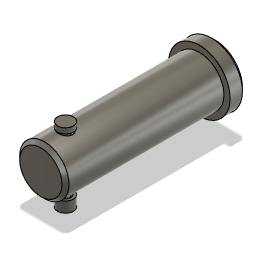
0.174.2818 - Axe d'articulation avec tête 14-45 type B (Autodesk Fusion 360 design; units mm, degrees)
Autodesk Fusion 360 part; units mm, degrees
sketch "Sketch1" plane through (0, 0, 0) normal (0, 0, 1) x (1, 0, 0)
  circle A0 centre (0, 0) radius 7
  dimension "d1" = 14
  constraint coincident A0.centre origin
  measures "d1" diameter of A0
extrude "Extrude1" add sketch "Sketch1" along normal blind 45 makes body 1
chamfer "Chamfer1" distance 1 angle 45 1 edges at (-6.5263, -2.5313, 45) on bodies 1
sketch "Sketch2" plane through (0, 0, 0) normal (0, 0, -1) x (-1, 0, 0)
  circle A0 centre (0, 0) radius 7
  circle A1 centre (0, 0) radius 8.75
  dimension "d5" = 17.5
  constraint coincident A0.centre A1.centre
  measures "d5" diameter of A1
extrude "Extrude2" add sketch "Sketch2" along normal blind 4.5 contours A0 | A1 bodies 1
chamfer "Chamfer2" distance 1 angle 45 1 edges at (8.1579, -3.1641, -4.5) on bodies 1
sketch "Sketch3" plane through (0, 0, 0) normal (0, 1, 0) x (1, 0, 0)
  line L0 (-7, -44) -> (7, -44) construction
  line L1 (-7, -38) -> (7, -38) construction
  line L2 (0, -44) -> (0, -38) construction
  circle A0 centre (0, -38) radius 2
  dimension "d9" = 6
  dimension "d10" = 4
  constraint midpoint L0 L2.start
  constraint midpoint L1 L2.end
  constraint perpendicular L1 L2
  constraint coincident L2.end A0.centre
  measures "d10" diameter of A0
extrude "Extrude3" cut sketch "Sketch3" along normal through all and the other way through all bodies 1
sketch "Sketch4" plane through (0, 0, 0) normal (0, 1, 0) x (1, 0, 0)
  spline S0 degree 3 poles (1.5, -38) (1.5, -37.8138) (1.4604, -37.6052) (1.385, -37.424) (1.3095, -37.2425) (1.1904, -37.0691) (1.0607, -36.9393) (0.931, -36.8096) (0.7575, -36.6905) (0.576, -36.615) (0.3947, -36.5396) (0.186, -36.5) (0, -36.5) (-0.186, -36.5) (-0.3947, -36.5396) (-0.576, -36.615) (-0.7575, -36.6905) (-0.931, -36.8096) (-1.0607, -36.9393) (-1.1904, -37.0691) (-1.3095, -37.2425) (-1.385, -37.424) (-1.4604, -37.6052) (-1.5, -37.8138) (-1.5, -38) (-1.5, -38.1862) (-1.4604, -38.3948) (-1.385, -38.576) (-1.3095, -38.7575) (-1.1904, -38.9309) (-1.0607, -39.0607) (-0.931, -39.1904) (-0.7575, -39.3095) (-0.576, -39.385) (-0.3947, -39.4604) (-0.186, -39.5) (0, -39.5) (0.186, -39.5) (0.3947, -39.4604) (0.576, -39.385) (0.7575, -39.3095) (0.931, -39.1904) (1.0607, -39.0607) (1.1904, -38.9309) (1.3095, -38.7575) (1.385, -38.576) (1.4604, -38.3948) (1.5, -38.1862) (1.5, -38) knots 0.60776 0.60776 0.60776 0.60776 0.683748 0.683748 0.683748 0.759735 0.759735 0.759735 0.835688 0.835688 0.835688 0.91164 0.91164 0.91164 0.987593 0.987593 0.987593 1.063545 1.063545 1.063545 1.139533 1.139533 1.139533 1.21552 1.21552 1.21552 1.291508 1.291508 1.291508 1.367496 1.367496 1.367496 1.443448 1.443448 1.443448 1.5194 1.5194 1.5194 1.595353 1.595353 1.595353 1.671305 1.671305 1.671305 1.747293 1.747293 1.747293 1.82328 1.82328 1.82328 1.82328
  spline S1 degree 3 poles (-2, -38) (-2, -37.7473) (-1.9492, -37.4788) (-1.7447, -36.9865) (-1.591, -36.7626) (-1.2375, -36.409) (-1.0135, -36.2553) (-0.5211, -36.0508) (-0.2526, -36) (0.2526, -36) (0.5211, -36.0508) (1.0135, -36.2553) (1.2375, -36.409) (1.591, -36.7626) (1.7447, -36.9865) (1.9492, -37.4788) (2, -37.7473) (2, -38.2527) (1.9492, -38.5212) (1.7447, -39.0135) (1.591, -39.2374) (1.2375, -39.591) (1.0135, -39.7447) (0.5211, -39.9492) (0.2526, -40) (-0.2526, -40) (-0.5211, -39.9492) (-1.0135, -39.7447) (-1.2375, -39.591) (-1.591, -39.2374) (-1.7447, -39.0135) (-1.9492, -38.5212) (-2, -38.2527) (-2, -38) knots 0 0 0 0 0.075804 0.075804 0.151609 0.151609 0.227394 0.227394 0.30318 0.30318 0.378966 0.378966 0.454752 0.454752 0.530556 0.530556 0.60636 0.60636 0.682165 0.682165 0.757969 0.757969 0.833755 0.833755 0.909541 0.909541 0.985326 0.985326 1.061112 1.061112 1.136916 1.136916 1.212721 1.212721 1.212721 1.212721
  line L0 (0, -68) -> (8.4815, -68)
  constraint horizontal L0
extrude "Extrude4" add sketch "Sketch4" along normal blind 9 and the other way blind 12 separate body contours S0 makes body 2
sketch "Sketch5" plane through (0, 9, 0) normal (0, 1, 0) x (-1, 0, 0)
  spline S0 degree 3 poles (1.5, -38) (1.5, -37.8138) (1.4604, -37.6052) (1.385, -37.424) (1.3095, -37.2425) (1.1904, -37.0691) (1.0607, -36.9393) (0.931, -36.8096) (0.7575, -36.6905) (0.576, -36.615) (0.3947, -36.5396) (0.186, -36.5) (0, -36.5) (-0.186, -36.5) (-0.3947, -36.5396) (-0.576, -36.615) (-0.7575, -36.6905) (-0.931, -36.8096) (-1.0607, -36.9393) (-1.1904, -37.0691) (-1.3095, -37.2425) (-1.385, -37.424) (-1.4604, -37.6052) (-1.5, -37.8138) (-1.5, -38) (-1.5, -38.1862) (-1.4604, -38.3948) (-1.385, -38.576) (-1.3095, -38.7575) (-1.1904, -38.9309) (-1.0607, -39.0607) (-0.931, -39.1904) (-0.7575, -39.3095) (-0.576, -39.385) (-0.3947, -39.4604) (-0.186, -39.5) (0, -39.5) (0.186, -39.5) (0.3947, -39.4604) (0.576, -39.385) (0.7575, -39.3095) (0.931, -39.1904) (1.0607, -39.0607) (1.1904, -38.9309) (1.3095, -38.7575) (1.385, -38.576) (1.4604, -38.3948) (1.5, -38.1862) (1.5, -38) knots 0.60776 0.60776 0.60776 0.60776 0.683748 0.683748 0.683748 0.759735 0.759735 0.759735 0.835688 0.835688 0.835688 0.91164 0.91164 0.91164 0.987593 0.987593 0.987593 1.063545 1.063545 1.063545 1.139533 1.139533 1.139533 1.21552 1.21552 1.21552 1.291508 1.291508 1.291508 1.367496 1.367496 1.367496 1.443448 1.443448 1.443448 1.5194 1.5194 1.5194 1.595353 1.595353 1.595353 1.671305 1.671305 1.671305 1.747293 1.747293 1.747293 1.82328 1.82328 1.82328 1.82328
  spline S1 degree 3 poles (-1.5, 38) (-1.5, 37.8138) (-1.4604, 37.6052) (-1.385, 37.424) (-1.3095, 37.2425) (-1.1904, 37.0691) (-1.0607, 36.9393) (-0.931, 36.8096) (-0.7575, 36.6905) (-0.576, 36.615) (-0.3947, 36.5396) (-0.186, 36.5) (0, 36.5) (0.186, 36.5) (0.3947, 36.5396) (0.576, 36.615) (0.7575, 36.6905) (0.931, 36.8096) (1.0607, 36.9393) (1.1904, 37.0691) (1.3095, 37.2425) (1.385, 37.424) (1.4604, 37.6052) (1.5, 37.8138) (1.5, 38) (1.5, 38.1862) (1.4604, 38.3948) (1.385, 38.576) (1.3095, 38.7575) (1.1904, 38.9309) (1.0607, 39.0607) (0.931, 39.1904) (0.7575, 39.3095) (0.576, 39.385) (0.3947, 39.4604) (0.186, 39.5) (0, 39.5) (-0.186, 39.5) (-0.3947, 39.4604) (-0.576, 39.385) (-0.7575, 39.3095) (-0.931, 39.1904) (-1.0607, 39.0607) (-1.1904, 38.9309) (-1.3095, 38.7575) (-1.385, 38.576) (-1.4604, 38.3948) (-1.5, 38.1862) (-1.5, 38) knots 0.60776 0.60776 0.60776 0.60776 0.683748 0.683748 0.683748 0.759735 0.759735 0.759735 0.835688 0.835688 0.835688 0.91164 0.91164 0.91164 0.987593 0.987593 0.987593 1.063545 1.063545 1.063545 1.139533 1.139533 1.139533 1.21552 1.21552 1.21552 1.291508 1.291508 1.291508 1.367496 1.367496 1.367496 1.443448 1.443448 1.443448 1.5194 1.5194 1.5194 1.595353 1.595353 1.595353 1.671305 1.671305 1.671305 1.747293 1.747293 1.747293 1.82328 1.82328 1.82328 1.82328 construction
  spline S2 degree 3 poles (-1.5, 38) (-1.5, 38.1862) (-1.4604, 38.3948) (-1.385, 38.576) (-1.3095, 38.7575) (-1.1904, 38.9309) (-1.0607, 39.0607) (-0.931, 39.1904) (-0.7575, 39.3095) (-0.576, 39.385) (-0.3947, 39.4604) (-0.186, 39.5) (0, 39.5) (0.186, 39.5) (0.3947, 39.4604) (0.576, 39.385) (0.7575, 39.3095) (0.931, 39.1904) (1.0607, 39.0607) (1.1904, 38.9309) (1.3095, 38.7575) (1.385, 38.576) (1.4604, 38.3948) (1.5, 38.1862) (1.5, 38) (1.5, 37.8138) (1.4604, 37.6052) (1.385, 37.424) (1.3095, 37.2425) (1.1904, 37.0691) (1.0607, 36.9393) (0.931, 36.8096) (0.7575, 36.6905) (0.576, 36.615) (0.3947, 36.5396) (0.186, 36.5) (0, 36.5) (-0.186, 36.5) (-0.3947, 36.5396) (-0.576, 36.615) (-0.7575, 36.6905) (-0.931, 36.8096) (-1.0607, 36.9393) (-1.1904, 37.0691) (-1.3095, 37.2425) (-1.385, 37.424) (-1.4604, 37.6052) (-1.5, 37.8138) (-1.5, 38) knots -1.82328 -1.82328 -1.82328 -1.82328 -1.747293 -1.747293 -1.747293 -1.671305 -1.671305 -1.671305 -1.595353 -1.595353 -1.595353 -1.5194 -1.5194 -1.5194 -1.443448 -1.443448 -1.443448 -1.367496 -1.367496 -1.367496 -1.291508 -1.291508 -1.291508 -1.21552 -1.21552 -1.21552 -1.139533 -1.139533 -1.139533 -1.063545 -1.063545 -1.063545 -0.987593 -0.987593 -0.987593 -0.91164 -0.91164 -0.91164 -0.835688 -0.835688 -0.835688 -0.759735 -0.759735 -0.759735 -0.683748 -0.683748 -0.683748 -0.60776 -0.60776 -0.60776 -0.60776 construction
  circle A0 centre (0, 38) radius 2.25
  spline S3 degree 3 poles (-2, -38) (-2, -37.7473) (-1.9492, -37.4788) (-1.7447, -36.9865) (-1.591, -36.7626) (-1.2375, -36.409) (-1.0135, -36.2553) (-0.5211, -36.0508) (-0.2526, -36) (0.2526, -36) (0.5211, -36.0508) (1.0135, -36.2553) (1.2375, -36.409) (1.591, -36.7626) (1.7447, -36.9865) (1.9492, -37.4788) (2, -37.7473) (2, -38.2527) (1.9492, -38.5212) (1.7447, -39.0135) (1.591, -39.2374) (1.2375, -39.591) (1.0135, -39.7447) (0.5211, -39.9492) (0.2526, -40) (-0.2526, -40) (-0.5211, -39.9492) (-1.0135, -39.7447) (-1.2375, -39.591) (-1.591, -39.2374) (-1.7447, -39.0135) (-1.9492, -38.5212) (-2, -38.2527) (-2, -38) knots 0 0 0 0 0.075804 0.075804 0.151609 0.151609 0.227394 0.227394 0.30318 0.30318 0.378966 0.378966 0.454752 0.454752 0.530556 0.530556 0.60636 0.60636 0.682165 0.682165 0.757969 0.757969 0.833755 0.833755 0.909541 0.909541 0.985326 0.985326 1.061112 1.061112 1.136916 1.136916 1.212721 1.212721 1.212721 1.212721
  spline S4 degree 3 poles (1.5, 38) (1.4997, 38.0291) (1.499, 38.0582) (1.4876, 38.2407) (1.4443, 38.4464) (1.2744, 38.8221) (1.1579, 38.9635) (1.0607, 39.0607) (0.9778, 39.1435) (0.881, 39.2184) (0.6163, 39.3807) (0.5167, 39.4099) (0.2655, 39.4873) (0.0596, 39.5123) (-0.2987, 39.4775) (-0.5139, 39.4246) (-0.8641, 39.2393) (-1.0281, 39.1108) (-1.2584, 38.8304) (-1.3708, 38.6429) (-1.4869, 38.2672) (-1.5123, 38.0612) (-1.478, 37.7046) (-1.4256, 37.4888) (-1.2414, 37.1391) (-1.1133, 36.9745) (-0.8077, 36.7224) (-0.6295, 36.6258) (-0.2761, 36.5151) (-0.0693, 36.488) (0.2839, 36.5201) (0.5004, 36.5708) (0.8431, 36.7475) (1.0118, 36.8739) (1.2827, 37.1947) (1.368, 37.3621) (1.4579, 37.6311) (1.4977, 37.8165) (1.5, 38) knots -0.080744 -0.080744 -0.080744 -0.080744 -0.074519 -0.074519 -0.041241 -0.041241 0 0 0 0.035143 0.035143 0.092639 0.092639 0.246463 0.246463 0.37223 0.37223 0.489793 0.489793 0.586811 0.586811 0.67816 0.67816 0.752062 0.752062 0.820566 0.820566 0.888592 0.888592 0.958337 0.958337 1.013363 1.013363 1.062684 1.062684 1.116599 1.116599 1.155794 1.155794 1.155794 1.155794
  spline S5 degree 3 poles (2, 38) (2, 37.7473) (1.9492, 37.4788) (1.7447, 36.9865) (1.591, 36.7626) (1.2375, 36.409) (1.0135, 36.2553) (0.5211, 36.0508) (0.2526, 36) (-0.2526, 36) (-0.5211, 36.0508) (-1.0135, 36.2553) (-1.2375, 36.409) (-1.591, 36.7626) (-1.7447, 36.9865) (-1.9492, 37.4788) (-2, 37.7473) (-2, 38) (-2, 38.2527) (-1.9492, 38.5212) (-1.7447, 39.0135) (-1.591, 39.2374) (-1.2375, 39.591) (-1.0135, 39.7447) (-0.5211, 39.9492) (-0.2526, 40) (0.2526, 40) (0.5211, 39.9492) (1.0135, 39.7447) (1.2375, 39.591) (1.591, 39.2374) (1.7447, 39.0135) (1.9492, 38.5212) (2, 38.2527) (2, 38) knots 0.60636 0.60636 0.60636 0.60636 0.682165 0.682165 0.757969 0.757969 0.833755 0.833755 0.909541 0.909541 0.985326 0.985326 1.061112 1.061112 1.136916 1.136916 1.212721 1.212721 1.212721 1.288525 1.288525 1.364329 1.364329 1.440115 1.440115 1.515901 1.515901 1.591687 1.591687 1.667473 1.667473 1.743277 1.743277 1.819081 1.819081 1.819081 1.819081
  spline S6 degree 3 poles (-2, 38) (-2, 37.7473) (-1.9492, 37.4788) (-1.7447, 36.9865) (-1.591, 36.7626) (-1.2375, 36.409) (-1.0135, 36.2553) (-0.5211, 36.0508) (-0.2526, 36) (0.2526, 36) (0.5211, 36.0508) (1.0135, 36.2553) (1.2375, 36.409) (1.591, 36.7626) (1.7447, 36.9865) (1.9492, 37.4788) (2, 37.7473) (2, 38.2527) (1.9492, 38.5212) (1.7447, 39.0135) (1.591, 39.2374) (1.2375, 39.591) (1.0135, 39.7447) (0.5211, 39.9492) (0.2526, 40) (-0.2526, 40) (-0.5211, 39.9492) (-1.0135, 39.7447) (-1.2375, 39.591) (-1.591, 39.2374) (-1.7447, 39.0135) (-1.9492, 38.5212) (-2, 38.2527) (-2, 38) knots 0 0 0 0 0.075804 0.075804 0.151609 0.151609 0.227394 0.227394 0.30318 0.30318 0.378966 0.378966 0.454752 0.454752 0.530556 0.530556 0.60636 0.60636 0.682165 0.682165 0.757969 0.757969 0.833755 0.833755 0.909541 0.909541 0.985326 0.985326 1.061112 1.061112 1.136916 1.136916 1.212721 1.212721 1.212721 1.212721
  dimension "d18" = 4.5
  measures "d18" diameter of A0
extrude "Extrude5" add sketch "Sketch5" against normal blind 1.5 contours A0 | S4 | S5 S6 bodies 2
sketch "Sketch6" plane through (0, -12, 0) normal (0, -1, 0) x (1, 0, 0)
  spline S0 degree 3 poles (1.5, 38) (1.5, 38.1862) (1.4604, 38.3948) (1.385, 38.576) (1.3095, 38.7575) (1.1904, 38.9309) (1.0607, 39.0607) (0.931, 39.1904) (0.7575, 39.3095) (0.576, 39.385) (0.3947, 39.4604) (0.186, 39.5) (0, 39.5) (-0.186, 39.5) (-0.3947, 39.4604) (-0.576, 39.385) (-0.7575, 39.3095) (-0.931, 39.1904) (-1.0607, 39.0607) (-1.1904, 38.9309) (-1.3095, 38.7575) (-1.385, 38.576) (-1.4604, 38.3948) (-1.5, 38.1862) (-1.5, 38) (-1.5, 37.8138) (-1.4604, 37.6052) (-1.385, 37.424) (-1.3095, 37.2425) (-1.1904, 37.0691) (-1.0607, 36.9393) (-0.931, 36.8096) (-0.7575, 36.6905) (-0.576, 36.615) (-0.3947, 36.5396) (-0.186, 36.5) (0, 36.5) (0.186, 36.5) (0.3947, 36.5396) (0.576, 36.615) (0.7575, 36.6905) (0.931, 36.8096) (1.0607, 36.9393) (1.1904, 37.0691) (1.3095, 37.2425) (1.385, 37.424) (1.4604, 37.6052) (1.5, 37.8138) (1.5, 38) knots -1.82328 -1.82328 -1.82328 -1.82328 -1.747293 -1.747293 -1.747293 -1.671305 -1.671305 -1.671305 -1.595353 -1.595353 -1.595353 -1.5194 -1.5194 -1.5194 -1.443448 -1.443448 -1.443448 -1.367496 -1.367496 -1.367496 -1.291508 -1.291508 -1.291508 -1.21552 -1.21552 -1.21552 -1.139533 -1.139533 -1.139533 -1.063545 -1.063545 -1.063545 -0.987593 -0.987593 -0.987593 -0.91164 -0.91164 -0.91164 -0.835688 -0.835688 -0.835688 -0.759735 -0.759735 -0.759735 -0.683748 -0.683748 -0.683748 -0.60776 -0.60776 -0.60776 -0.60776 construction
  spline S1 degree 3 poles (1.5, 38) (1.5, 38.1862) (1.4604, 38.3948) (1.385, 38.576) (1.3095, 38.7575) (1.1904, 38.9309) (1.0607, 39.0607) (0.931, 39.1904) (0.7575, 39.3095) (0.576, 39.385) (0.3947, 39.4604) (0.186, 39.5) (0, 39.5) (-0.186, 39.5) (-0.3947, 39.4604) (-0.576, 39.385) (-0.7575, 39.3095) (-0.931, 39.1904) (-1.0607, 39.0607) (-1.1904, 38.9309) (-1.3095, 38.7575) (-1.385, 38.576) (-1.4604, 38.3948) (-1.5, 38.1862) (-1.5, 38) (-1.5, 37.8138) (-1.4604, 37.6052) (-1.385, 37.424) (-1.3095, 37.2425) (-1.1904, 37.0691) (-1.0607, 36.9393) (-0.931, 36.8096) (-0.7575, 36.6905) (-0.576, 36.615) (-0.3947, 36.5396) (-0.186, 36.5) (0, 36.5) (0.186, 36.5) (0.3947, 36.5396) (0.576, 36.615) (0.7575, 36.6905) (0.931, 36.8096) (1.0607, 36.9393) (1.1904, 37.0691) (1.3095, 37.2425) (1.385, 37.424) (1.4604, 37.6052) (1.5, 37.8138) (1.5, 38) knots -1.82328 -1.82328 -1.82328 -1.82328 -1.747293 -1.747293 -1.747293 -1.671305 -1.671305 -1.671305 -1.595353 -1.595353 -1.595353 -1.5194 -1.5194 -1.5194 -1.443448 -1.443448 -1.443448 -1.367496 -1.367496 -1.367496 -1.291508 -1.291508 -1.291508 -1.21552 -1.21552 -1.21552 -1.139533 -1.139533 -1.139533 -1.063545 -1.063545 -1.063545 -0.987593 -0.987593 -0.987593 -0.91164 -0.91164 -0.91164 -0.835688 -0.835688 -0.835688 -0.759735 -0.759735 -0.759735 -0.683748 -0.683748 -0.683748 -0.60776 -0.60776 -0.60776 -0.60776 construction
  circle A0 centre (0, 38) radius 2.25
  spline S2 degree 3 poles (1.5, 38) (1.4997, 38.0291) (1.499, 38.0582) (1.4876, 38.2407) (1.4443, 38.4464) (1.2744, 38.8221) (1.1579, 38.9635) (1.0607, 39.0607) (0.9778, 39.1435) (0.881, 39.2184) (0.6163, 39.3807) (0.5167, 39.4099) (0.2655, 39.4873) (0.0596, 39.5123) (-0.2987, 39.4775) (-0.5139, 39.4246) (-0.8641, 39.2393) (-1.0281, 39.1108) (-1.2584, 38.8304) (-1.3708, 38.6429) (-1.4869, 38.2672) (-1.5123, 38.0612) (-1.478, 37.7046) (-1.4256, 37.4888) (-1.2414, 37.1391) (-1.1133, 36.9745) (-0.8077, 36.7224) (-0.6295, 36.6258) (-0.2761, 36.5151) (-0.0693, 36.488) (0.2839, 36.5201) (0.5004, 36.5708) (0.8431, 36.7475) (1.0118, 36.8739) (1.2827, 37.1947) (1.368, 37.3621) (1.4579, 37.6311) (1.4977, 37.8165) (1.5, 38) knots -0.080744 -0.080744 -0.080744 -0.080744 -0.074519 -0.074519 -0.041241 -0.041241 0 0 0 0.035143 0.035143 0.092639 0.092639 0.246463 0.246463 0.37223 0.37223 0.489793 0.489793 0.586811 0.586811 0.67816 0.67816 0.752062 0.752062 0.820566 0.820566 0.888592 0.888592 0.958337 0.958337 1.013363 1.013363 1.062684 1.062684 1.116599 1.116599 1.155794 1.155794 1.155794 1.155794
  spline S3 degree 3 poles (2, 38) (2, 37.7473) (1.9492, 37.4788) (1.7447, 36.9865) (1.591, 36.7626) (1.2375, 36.409) (1.0135, 36.2553) (0.5211, 36.0508) (0.2526, 36) (-0.2526, 36) (-0.5211, 36.0508) (-1.0135, 36.2553) (-1.2375, 36.409) (-1.591, 36.7626) (-1.7447, 36.9865) (-1.9492, 37.4788) (-2, 37.7473) (-2, 38) (-2, 38.2527) (-1.9492, 38.5212) (-1.7447, 39.0135) (-1.591, 39.2374) (-1.2375, 39.591) (-1.0135, 39.7447) (-0.5211, 39.9492) (-0.2526, 40) (0.2526, 40) (0.5211, 39.9492) (1.0135, 39.7447) (1.2375, 39.591) (1.591, 39.2374) (1.7447, 39.0135) (1.9492, 38.5212) (2, 38.2527) (2, 38) knots 0.60636 0.60636 0.60636 0.60636 0.682165 0.682165 0.757969 0.757969 0.833755 0.833755 0.909541 0.909541 0.985326 0.985326 1.061112 1.061112 1.136916 1.136916 1.212721 1.212721 1.212721 1.288525 1.288525 1.364329 1.364329 1.440115 1.440115 1.515901 1.515901 1.591687 1.591687 1.667473 1.667473 1.743277 1.743277 1.819081 1.819081 1.819081 1.819081
  spline S4 degree 3 poles (-2, 38) (-2, 37.7473) (-1.9492, 37.4788) (-1.7447, 36.9865) (-1.591, 36.7626) (-1.2375, 36.409) (-1.0135, 36.2553) (-0.5211, 36.0508) (-0.2526, 36) (0.2526, 36) (0.5211, 36.0508) (1.0135, 36.2553) (1.2375, 36.409) (1.591, 36.7626) (1.7447, 36.9865) (1.9492, 37.4788) (2, 37.7473) (2, 38.2527) (1.9492, 38.5212) (1.7447, 39.0135) (1.591, 39.2374) (1.2375, 39.591) (1.0135, 39.7447) (0.5211, 39.9492) (0.2526, 40) (-0.2526, 40) (-0.5211, 39.9492) (-1.0135, 39.7447) (-1.2375, 39.591) (-1.591, 39.2374) (-1.7447, 39.0135) (-1.9492, 38.5212) (-2, 38.2527) (-2, 38) knots 0 0 0 0 0.075804 0.075804 0.151609 0.151609 0.227394 0.227394 0.30318 0.30318 0.378966 0.378966 0.454752 0.454752 0.530556 0.530556 0.60636 0.60636 0.682165 0.682165 0.757969 0.757969 0.833755 0.833755 0.909541 0.909541 0.985326 0.985326 1.061112 1.061112 1.136916 1.136916 1.212721 1.212721 1.212721 1.212721
  point P0 (1.5, 38)
  dimension "d21" = 4.5
  measures "d21" diameter of A0
extrude "Extrude6" add sketch "Sketch6" against normal blind 3 contours A0 | S2 | S3 S4 bodies 2
